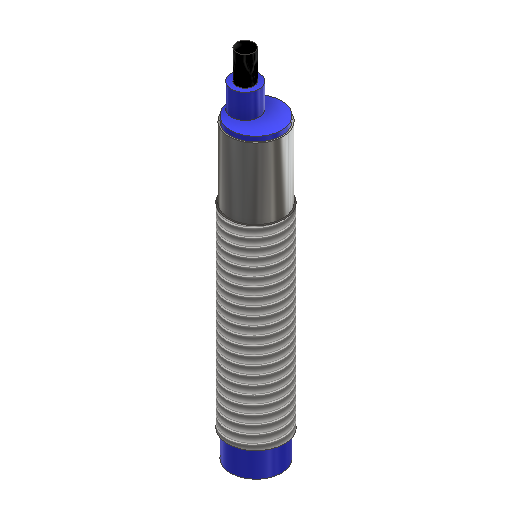
# Autodesk Inventor part: COTS_GENERIC_Induction_Distance_Sensor
Saved by Autodesk Inventor 2026.1 (Build 301233000, 233)
## iProperties
Created: 2017-05-27
Part Number: COTS_GENERIC_Induction_Distance_Sensor
Material: Ogólny
Document SubType Name: Modeling
Designer: Andrzej
Density: 1 g/cm^3
Appearance: Stal - polerowana
Mass: 6.45517 g
Surface Area: 25.6274 cm^2
Volume: 6.45517 cm^3
Author: Andrzej
Autodesk Inventor part; units mm, degrees
ref_plane "YZ Plane" through (0, 0, 0) normal (1, 0, 0) x (0, 1, 0)
ref_plane "XZ Plane" through (0, 0, 0) normal (0, 1, 0) x (-1, 0, 0)
ref_plane "XY Plane" through (0, 0, 0) normal (0, 0, 1) x (1, 0, 0)
sketch "Szkic1" plane through (0, 0, 0) normal (0, 0, 1) x (1, 0, 0)
  circle A0 centre (0, 0) radius 5.25
  dimension "d0" = 10.5
  constraints: 1 centre point, 1 coincident
  measures "d0" diameter of A0
extrude "Wyciągnięcie proste1" add sketch "Szkic1" along normal blind 5.5
sketch "Szkic2" plane through (0, 0, 5.5) normal (0, 0, 1) x (1, 0, 0)
  circle A0 centre (0, 0) radius 5.25 projected
  circle A1 centre (0, 0) radius 5.85
  dimension "d3" = 11.7
  constraints: 1 centre point, 1 coincident
  measures "d3" diameter of A1
extrude "Wyciągnięcie proste2" add sketch "Szkic2" along normal blind 40 contours A0 | A1
sketch "Szkic3" plane through (0, 0, 45.5) normal (0, 0, 1) x (1, 0, 0)
  circle A0 centre (0, 0) radius 5.85 projected
  circle A1 centre (0, 0) radius 5.55
  dimension "d6" = 11.1
  constraints: 1 centre point, 1 coincident
  measures "d6" diameter of A1
extrude "Wyciągnięcie proste3" add sketch "Szkic3" along normal blind 14.5 contours A1
thread "Gwint1" size "M12x1.75" class "6g" standard "ANSI Metric M Profile" full length
sketch "Szkic4" plane through (0, 0, 60) normal (0, 0, 1) x (1, 0, 0)
  circle A0 centre (0, 0) radius 5.25
  dimension "d11" = 10.5
  constraints: 1 centre point, 1 coincident
  measures "d11" diameter of A0
extrude "Wyciągnięcie proste4" add sketch "Szkic4" along normal blind 1
sketch "Szkic5" plane through (0, 0, 61) normal (0, 0, 1) x (1, 0, 0)
  circle A0 centre (0, 0) radius 5.25 projected
  circle A1 centre (-2.2069, 0) radius 2.85
  dimension "d14" = 5.7
  constraints: 1 centre point
  measures "d14" diameter of A1
extrude "Wyciągnięcie proste5" add sketch "Szkic5" along normal blind 5 contours A1
sketch "Szkic6" plane through (-2.2069, 0, 66) normal (0, 0, 1) x (1, 0, 0)
  circle A0 centre (0, 0) radius 2.85 projected
  circle A1 centre (0, 0) radius 1.8
  point P0 (2.2069, 0)
  dimension "d17" = 3.6
  constraints: 1 centre point, 1 coincident
  measures "d17" diameter of A1
extrude "Wyciągnięcie proste6" add sketch "Szkic6" along normal blind 6 contours A1
